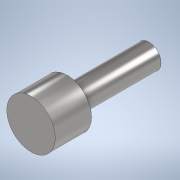
# Autodesk Inventor part: 5mm_bolt_short
Saved by Autodesk Inventor 2021.2 (Build 252289000, 289)
## iProperties
Created: 2021-02-17
Part Number: 5mm_bolt_short
Material: Steel, Alloy
Document SubType Name: Modeling
Designer: yxion
Density: 7.73 g/cm^3
Appearance: Semi-Polished
Author: yxion
Autodesk Inventor part; units mm, degrees
ref_plane "YZ Plane" through (0, 0, 0) normal (1, 0, 0) x (0, 1, 0)
ref_plane "XZ Plane" through (0, 0, 0) normal (0, 1, 0) x (-1, 0, 0)
ref_plane "XY Plane" through (0, 0, 0) normal (0, 0, 1) x (1, 0, 0)
sketch "Sketch1" plane through (0, 0, 0) normal (0, 0, 1) x (1, 0, 0)
  circle A0 centre (0.8326, 3.0356) radius 2.5
  point P0 (0, 0)
  dimension "d0" = 5
  constraints: 1 centre point
  measures "d0" diameter of A0
extrude "Extrusion1" add sketch "Sketch1" along normal blind 29.972
sketch "Sketch2" plane through (0.8326, 3.0356, 29.972) normal (0, 0, 1) x (1, 0, 0)
  circle A0 centre (0, 0) radius 2.5 projected
  circle A1 centre (0, 0) radius 5.015
  point P0 (-0.8326, -3.0356)
  constraints: 1 centre point
extrude "Extrusion2" add sketch "Sketch2" along normal blind 7.5 contours A0 | A1
sketch "Sketch3" plane through (0.8326, 3.0356, 0) normal (0, 0, -1) x (-1, 0, 0)
  circle A0 centre (0, 0) radius 5.015 projected
  circle A1 centre (0, 0) radius 2.5 projected
  circle A2 centre (0, 0) radius 2.5 projected
  point P0 (0.8326, -3.0356)
extrude "Extrusion3" add sketch "Sketch3" along normal blind 6 contours A1
sketch "Sketch4" plane through (0.8326, 3.0356, -6) normal (0, 0, -1) x (-1, 0, 0)
  circle A0 centre (0, 0) radius 2.5 projected
  point P0 (0.8326, -3.0356)
extrude "Extrusion4" cut sketch "Sketch4" against normal blind 19.05
body "Solid1"
